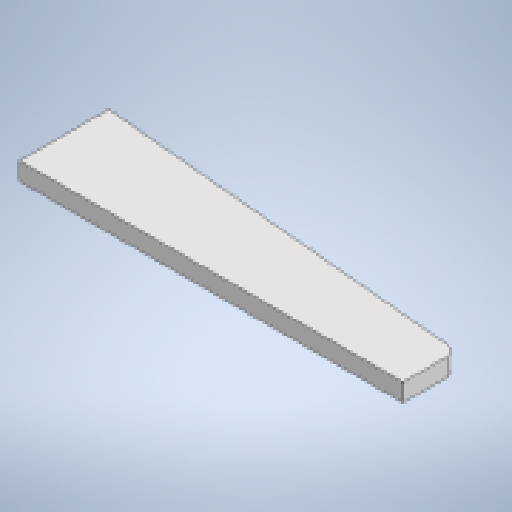
# Autodesk Inventor part: PRS 940-24 charging hatch reinf 500mm
Saved by Autodesk Inventor 2025.4 (Build 294407000, 407)
## iProperties
Created: 2025-02-12
Part Number: PRS 940-24 charging hatch reinf 500mm
Material: Steel
Document SubType Name: Sheet Metal
Designer: user
Density: 7.85 g/cm^3
Flat Pattern Width: 4.99208 cm
Flat Pattern Length: 21.7472 cm
Flat Pattern Area: 108.564 cm^2
Sheet Metal Rule: Default_mm
Sheet Metal Width: 49,921 mm
Sheet Metal Length: 217,472 mm
Sheet Metal Area: 10856,387 mm^2
Appearance: Default
Author: pokla
Autodesk Inventor part; units mm, degrees
ref_plane "YZ Plane" through (0, 0, 0) normal (1, 0, 0) x (0, 1, 0)
ref_plane "XZ Plane" through (0, 0, 0) normal (0, 1, 0) x (-1, 0, 0)
ref_plane "XY Plane" through (0, 0, 0) normal (0, 0, 1) x (1, 0, 0)
sketch "Sketch3" plane through (0, 0, 0) normal (0, 0, 1) x (1, 0, 0)
  line L0 (0, 0) -> (260, 0)
  line L1 (260, 0) -> (260, 30)
  line L2 (260, 30) -> (-45.1628, 58.3872)
  line L3 (45, 50) -> (45, 0)
  dimension "d11" = 260
  dimension "d12" = 30
  dimension "d13" = 45
  dimension "d14" = 50
  measures "d11" distance of L0.start L0.end
  measures "d12" distance of L0.end L1.end
  measures "d13" distance from line of L0.start L3
  measures "d14" distance of L3.start L3.end
extrude "Plate1" add sketch "Sketch3" along normal mid plane 10
fillet "Corner Round1" radius 6 1 edges at (260, 30, 0)
equation "\"d15\" = Thickness"
equation "\"BendReliefDepth\" = 0.5 * Thickness"
equation "\"Thickness\" = 10"
body "Solid2"
